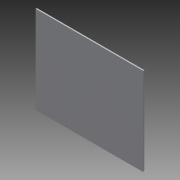
# Autodesk Inventor part: Plate_Top_Alu25
Saved by Autodesk Inventor 2013 (Build 170138000, 138)
## iProperties
Created: 2015-07-02
Part Number: Plate_Top_Alu25
Material: Aluminum 6061
Document SubType Name: Modeling
Designer: Kyle
Density: 2.71 g/cm^3
Mass: 21.5337 g
Surface Area: 199.36 cm^2
Volume: 7.94602 cm^3
Author: Kyle
Autodesk Inventor part; units mm, degrees
ref_plane "YZ Plane" through (0, 0, 0) normal (1, 0, 0) x (0, 1, 0)
ref_plane "XZ Plane" through (0, 0, 0) normal (0, 1, 0) x (-1, 0, 0)
ref_plane "XY Plane" through (0, 0, 0) normal (0, 0, 1) x (1, 0, 0)
sketch "Sketch1" plane through (0, 0, 0) normal (0, 0, 1) x (1, 0, 0)
  line L0 (0, 0) -> (109.22, 0)
  line L1 (109.22, 0) -> (109.22, 88.9)
  line L2 (109.22, 88.9) -> (0, 88.9)
  line L3 (0, 88.9) -> (0, 0)
  dimension "d0" = 109.22
  dimension "d1" = 88.9
  constraints: 8 end point, 2 parallel, 1 horizontal, 1 perpendicular
  measures "d0" distance of L1.end L2.end
  measures "d1" distance of L2.end L0.start
extrude "Extrusion1" add sketch "Sketch1" along normal blind 1.2903
chamfer "Chamfer1" distance 1.2903 angle 45 1 edges at (54.61, 0, 0)
body "Solid1"
